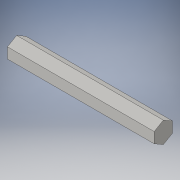
# Autodesk Inventor part: 3 Inch Hex Chafter
Saved by Autodesk Inventor 2016 (Build 200138000, 138)
## iProperties
Created: 2016-01-30
Part Number: 3 Inch Hex Chafter
Material: Generic
Document SubType Name: Modeling
Designer: gus
Density: 1 g/cm^3
Appearance: Default
Author: gus
Autodesk Inventor part; units mm, degrees
ref_plane "YZ Plane" through (0, 0, 0) normal (1, 0, 0) x (0, 1, 0)
ref_plane "XZ Plane" through (0, 0, 0) normal (0, 1, 0) x (-1, 0, 0)
ref_plane "XY Plane" through (0, 0, 0) normal (0, 0, 1) x (1, 0, 0)
sketch "Sketch1" plane through (0, 0, 0) normal (1, 0, 0) x (0, 1, 0)
  line L0 (-3.1315, -13.1005) -> (-8.6308, -13.1005)
  line L1 (-8.6308, -13.1005) -> (-11.3804, -8.338)
  line L2 (-11.3804, -8.338) -> (-8.6308, -3.5755)
  line L3 (-8.6308, -3.5755) -> (-3.1315, -3.5755)
  line L4 (-3.1315, -3.5755) -> (-0.3819, -8.338)
  line L5 (-0.3819, -8.338) -> (-3.1315, -13.1005)
  point P0 (0, 0)
  point P1 (-5.8811, -8.338)
  dimension "d0" = 9.525
  constraints: 12 end point, 1 horizontal, 13 other
  measures "d0" distance between parallel lines of L0 L3
extrude "Extrusion1" add sketch "Sketch1" along normal blind 76.2
body "Solid1"
